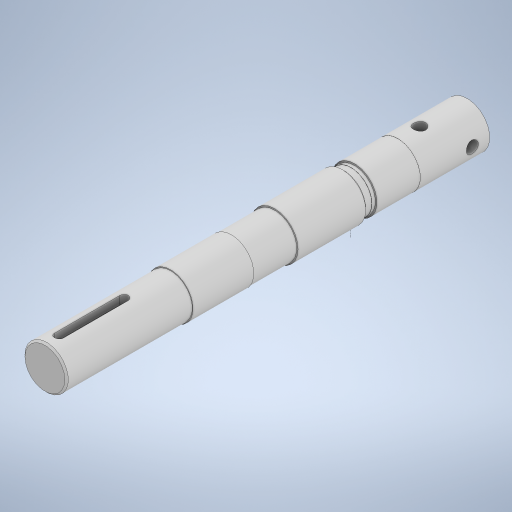
# Autodesk Inventor part: Mangon_Conduccion
Saved by Autodesk Inventor 2024 (Build 280153000, 153)
## iProperties
Created: 2026-01-05
Part Number: Mangon_Conduccion
Material: Generic
Document SubType Name: Modeling
Designer: eduso
Density: 1 g/cm^3
Appearance: Default
Testero_007: 4,000 mm
Espacio_008: 50,000 mm
Inteerior_Tubo_009: 80,000 mm
Author: eduso
Autodesk Inventor part; units mm, degrees
ref_plane "YZ Plane" through (0, 0, 0) normal (1, 0, 0) x (0, 1, 0)
ref_plane "XY Plane" through (0, 0, 0) normal (0, 0, 1) x (1, 0, 0)
sketch "Sketch1" plane through (0, 0, 0) normal (0, 1, 0) x (-1, 0, 0)
  line L0 (24, 8) -> (27, 8)
  line L1 (27, 8) -> (27, 88)
  line L2 (27, 88) -> (25.5, 88)
  line L3 (25.5, 88) -> (25.5, 138)
  line L4 (25.5, 138) -> (26, 138)
  line L5 (26, 138) -> (26, 208)
  line L6 (26, 208) -> (25, 208)
  line L7 (25, 208) -> (25, 248)
  line L8 (25, 248) -> (25, 248)
  line L9 (25, 248) -> (25, 353)
  line L10 (25, 353) -> (0, 353)
  line L11 (0, 189.8856) -> (0, -122.7414) construction
  line L12 (24, 8) -> (24, 0)
  line L13 (0, 353) -> (0, 0)
  line L14 (24, 0) -> (24.2, 0)
  line L15 (24.2, 0) -> (24.2, -4)
  line L16 (24.2, -4) -> (26, -4)
  line L17 (26, -4) -> (26, -54)
  line L18 (26, -54) -> (26.1, -54)
  line L19 (26.1, -54) -> (26.1, -134)
  line L20 (26.1, -134) -> (0, -134)
  line L21 (0, 0) -> (0, -134)
  line L22 (24, 0) -> (24.2, 0)
  dimension "d0" = 105
  dimension "d3" = 70
  dimension "d2" = 80
  dimension "d4" = 8
  dimension "d15" = 40
  dimension "d16" = 50
  dimension "d69" = 25
  dimension "d70" = 26
  dimension "d71" = 27
  dimension "d78" = 24
  dimension "d82" = 4
  dimension "d83" = 50
  dimension "d84" = 24.2
  dimension "d85" = 26.1
  dimension "d86" = 80
  dimension "d87" = 25
  dimension "d88" = 25.5
  dimension "d89" = 26
  constraints: 46 end point, 10 perpendicular, 3 horizontal, 3 vertical, 2 collinear, 1 point on line, 3 other
  measures "d0" distance of L8.end L9.end
  measures "d3" distance of L4.end L5.end
  measures "d2" distance of L0.end L1.end
  measures "d4" distance of L0.start L12.end
  measures "d15" distance of L6.end L7.end
  measures "d16" distance of L2.end L3.end
  measures "d69" distance between parallel lines of L13 L9
  measures "d70" distance between parallel lines of L13 L5
  measures "d71" distance between parallel lines of L1 L13
  measures "d78" distance between parallel lines of L11 L12
  measures "d82" distance of L14.end L15.end
  measures "d83" distance of L16.end L17.end
  measures "d84" distance between parallel lines of L11 L15
  measures "d85" distance between parallel lines of L21 L19
  measures "d86" distance of L18.end L19.end
  measures "d87" distance between parallel lines of L13 L7
  measures "d88" distance between parallel lines of L11 L3
  measures "d89" distance between parallel lines of L11 L17
ref_plane "Work Plane1" through (0, 15, 0) normal (0, 1, 0) x (-1, 0, 0)
sketch "Sketch2" plane through (0, 15, 0) normal (0, 1, 0) x (-1, 0, 0)
  arc A0 (-5, 262) -> (5, 262) centre (0, 262) ccw
  arc A1 (5, 337) -> (-5, 337) centre (0, 337) ccw
  line L0 (-5, 337) -> (-5, 262)
  line L1 (5, 337) -> (5, 262)
  line L2 (0, 0) -> (0, 401.4271) construction
  dimension "d18" = 10
  dimension "d19" = 10
  dimension "d65" = 262
  dimension "d68" = 75
  constraints: 6 end point, 4 point on circle, 3 tangent, 2 centre point, 2 point on line, 1 parallel, 1 vertical
  measures "d18" diameter of A0
  measures "d19" diameter of A1
  measures "d65" distance of L2.start A0.centre
  measures "d68" distance of A1.centre A0.centre
sketch "Sketch3" plane through (0, 15, 0) normal (0, 1, 0) x (-1, 0, 0)
  circle A0 centre (0, -79) radius 7
  point P0 (0, 0)
  dimension "d22" = 14
  dimension "d66" = 79
  constraints: 1 centre point
  measures "d22" diameter of A0
  measures "d66" distance of point (0, 0) A0.centre
sketch "Sketch4" plane through (0, 0, 0) normal (1, 0, 0) x (0, 1, 0)
  circle A0 centre (0, -114) radius 7
  point P0 (0, 0)
  dimension "d28" = 14
  dimension "d67" = 114
  constraints: 1 centre point
  measures "d28" diameter of A0
  measures "d67" distance of point (0, 0) A0.centre
revolve "Revolution1" add sketch "Sketch1" angle 360 about axis through (0, 0, 353) along (0, 0, -1)
extrude "Extrusion4" cut sketch "Sketch2" along normal blind 10
extrude "Extrusion5" cut sketch "Sketch3" along normal blind 20 and the other way blind 45
extrude "Extrusion6" cut sketch "Sketch4" along normal blind 35 and the other way blind 30
chamfer "Chamfer1" distance 2 angle 45 1 edges at (25, 0, 353)
chamfer "Chamfer3" distance 2 angle 45 1 edges at (27, 0, 8)
sketch "Sketch5" plane through (0, 0, 0) normal (0, 1, 0) x (-1, 0, 0)
  line L0 (24, 8) -> (24, 0) projected
  point P0 (0, 0)
sketch "Sketch6" plane through (0, 0, 0) normal (1, 0, 0) x (0, 1, 0)
  line L0 (0, 0) -> (-46.2751, 0) construction
  constraints: 2 end point, 1 horizontal
body "Solid4"
